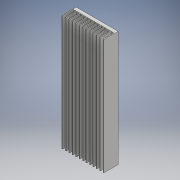
# Autodesk Inventor part: heat sink
Saved by Autodesk Inventor 2018 (Build 220112000, 112)
## iProperties
Created: 2018-06-04
Part Number: heat sink
Material: Generic
Document SubType Name: Modeling
Designer: John Viljoen
Density: 1 g/cm^3
Appearance: Default
Author: John Viljoen
Autodesk Inventor part; units mm, degrees
ref_plane "YZ Plane" through (0, 0, 0) normal (1, 0, 0) x (0, 1, 0)
ref_plane "XZ Plane" through (0, 0, 0) normal (0, 1, 0) x (-1, 0, 0)
ref_plane "XY Plane" through (0, 0, 0) normal (0, 0, 1) x (1, 0, 0)
sketch "Sketch4" plane through (0, 0, 0) normal (0, 0, 1) x (1, 0, 0)
  line L0 (0, 0) -> (97.04, 0)
  line L1 (97.04, 0) -> (97.04, 7.8)
  line L2 (97.04, 7.8) -> (0, 7.8)
  line L3 (0, 7.8) -> (0, 0)
  dimension "d15" = 97.04
  dimension "d16" = 7.8
  constraints: 8 end point, 2 horizontal, 2 perpendicular
  measures "d15" distance of L0.start L0.end
  measures "d16" distance of L0.end L1.end
extrude "Extrusion3" add sketch "Sketch4" along normal blind 267
sketch "Sketch5" plane through (0, 0, 267) normal (0, 0, 1) x (1, 0, 0)
  line L0 (0, 0) -> (97.04, 0) projected
  line L1 (0, 0) -> (1.8, 0)
  line L2 (1.8, 0) -> (1.8, -25.2)
  line L3 (1.8, -25.2) -> (0, -25.2)
  line L4 (0, -25.2) -> (0, 0)
  line L5 (9.7367, 0) -> (9.7367, -25.2)
  line L6 (7.9367, 0) -> (9.7367, 0)
  line L7 (7.9367, -25.2) -> (7.9367, 0)
  line L8 (9.7367, -25.2) -> (7.9367, -25.2)
  line L9 (17.6733, 0) -> (17.6733, -25.2)
  line L10 (15.8733, 0) -> (17.6733, 0)
  line L11 (15.8733, -25.2) -> (15.8733, 0)
  line L12 (17.6733, -25.2) -> (15.8733, -25.2)
  line L13 (25.61, 0) -> (25.61, -25.2)
  line L14 (23.81, 0) -> (25.61, 0)
  line L15 (23.81, -25.2) -> (23.81, 0)
  line L16 (25.61, -25.2) -> (23.81, -25.2)
  line L17 (33.5467, 0) -> (33.5467, -25.2)
  line L18 (31.7467, 0) -> (33.5467, 0)
  line L19 (31.7467, -25.2) -> (31.7467, 0)
  line L20 (33.5467, -25.2) -> (31.7467, -25.2)
  line L21 (41.4833, 0) -> (41.4833, -25.2)
  line L22 (39.6833, 0) -> (41.4833, 0)
  line L23 (39.6833, -25.2) -> (39.6833, 0)
  line L24 (41.4833, -25.2) -> (39.6833, -25.2)
  line L25 (49.42, 0) -> (49.42, -25.2)
  line L26 (47.62, 0) -> (49.42, 0)
  line L27 (47.62, -25.2) -> (47.62, 0)
  line L28 (49.42, -25.2) -> (47.62, -25.2)
  line L29 (57.3567, 0) -> (57.3567, -25.2)
  line L30 (55.5567, 0) -> (57.3567, 0)
  line L31 (55.5567, -25.2) -> (55.5567, 0)
  line L32 (57.3567, -25.2) -> (55.5567, -25.2)
  line L33 (65.2933, 0) -> (65.2933, -25.2)
  line L34 (63.4933, 0) -> (65.2933, 0)
  line L35 (63.4933, -25.2) -> (63.4933, 0)
  line L36 (65.2933, -25.2) -> (63.4933, -25.2)
  line L37 (73.23, 0) -> (73.23, -25.2)
  line L38 (71.43, 0) -> (73.23, 0)
  line L39 (71.43, -25.2) -> (71.43, 0)
  line L40 (73.23, -25.2) -> (71.43, -25.2)
  line L41 (81.1667, 0) -> (81.1667, -25.2)
  line L42 (79.3667, 0) -> (81.1667, 0)
  line L43 (79.3667, -25.2) -> (79.3667, 0)
  line L44 (81.1667, -25.2) -> (79.3667, -25.2)
  line L45 (89.1033, 0) -> (89.1033, -25.2)
  line L46 (87.3033, 0) -> (89.1033, 0)
  line L47 (87.3033, -25.2) -> (87.3033, 0)
  line L48 (89.1033, -25.2) -> (87.3033, -25.2)
  line L49 (97.04, 0) -> (97.04, -25.2)
  line L50 (95.24, 0) -> (97.04, 0)
  line L51 (95.24, -25.2) -> (95.24, 0)
  line L52 (97.04, -25.2) -> (95.24, -25.2)
  dimension "d19" = 1.8
  dimension "d20" = 25.2
  dimension "d23" = 7.9367
  constraints: 104 end point, 2 horizontal, 2 parallel, 1 perpendicular, 96 other
  measures "d19" distance of L2.end L3.end
  measures "d20" distance of L1.end L2.end
  measures "d23" distance of L1.end L5.start
extrude "Extrusion4" add sketch "Sketch5" against normal up to surface (267 mm away)
body "Solid2"
